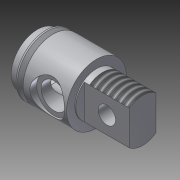
# Autodesk Inventor part: Rebuild Shooter NCDME075-0600 Cylinder Back Section
Saved by Autodesk Inventor 2014 SP1 (Build 180222100, 222)
## iProperties
Created: 2013-12-20
Part Number: Rebuild Shooter NCDME075-0600 Cylinder Back Section
Material: Aluminum 6061
Document SubType Name: Modeling
Designer: Moses
Mass: 18.68 g
Surface Area: 42.1842 cm^2
Volume: 6.893 cm^3
Density: 2.71 g/cm^3
Appearance: Aluminum - Flat
Author: Moses
Autodesk Inventor part; units mm, degrees
ref_plane "YZ Plane" through (0, 0, 0) normal (1, 0, 0) x (0, 1, 0)
ref_plane "XZ Plane" through (0, 0, 0) normal (0, 1, 0) x (-1, 0, 0)
sketch "Sketch1" plane through (0, 0, 0) normal (0, 0, 1) x (1, 0, 0)
  line L0 (0, 0) -> (35.3368, 0)
  line L1 (0, 10.922) -> (1.397, 9.525)
  line L2 (0, 10.922) -> (0.5388, 10.922)
  line L3 (0.5388, 10.922) -> (2.5708, 8.89)
  line L4 (2.5708, 8.89) -> (2.5708, 10.922)
  line L5 (2.5708, 10.922) -> (18.4458, 10.922)
  line L6 (18.4458, 10.922) -> (18.4458, 7.9248)
  line L7 (18.4458, 7.9248) -> (20.7318, 7.9248)
  line L8 (20.7318, 7.9248) -> (20.7318, 7.9375)
  line L9 (20.7318, 7.9375) -> (35.3368, 7.9375)
  line L10 (35.3368, 7.9375) -> (35.3368, 0)
  circle A0 centre (11.3338, 0) radius 4.7625
  circle A1 centre (27.0818, 0) radius 3.175
  line L11 (0, 10.922) -> (0, 0) construction
  line L12 (0.5388, 10.922) -> (2.5708, 10.922) construction
  line L13 (2.5708, 8.89) -> (2.5708, 7.9375) construction
  line L14 (1.397, 9.525) -> (0, 9.525)
  line L15 (0, 9.525) -> (0, 7.9375) construction
  line L16 (2.5708, 7.9375) -> (0, 7.9375)
  line L17 (0, 9.525) -> (0, 7.9375)
  line L18 (2.5708, 7.9375) -> (2.5708, 4.826)
  line L19 (2.5708, 4.826) -> (18.4458, 4.826)
  line L20 (18.4458, 4.826) -> (18.4458, 0)
  line L21 (18.4458, 7.9248) -> (18.4458, 4.826)
  line L22 (35.3368, 4.826) -> (18.4458, 4.826)
  line L23 (0, 9.525) -> (-3.175, 9.525)
  line L24 (-3.175, 9.525) -> (-3.175, 7.9375)
  line L25 (-3.175, 7.9375) -> (0, 7.9375)
  dimension "d1" = 21.844
  dimension "d2" = 9.525
  dimension "d4" = 2.286
  dimension "d5" = 6.35
  dimension "d6" = 8.636
  dimension "d8" = 15.8496
  dimension "d9" = 15.875
  dimension "d10" = 0.381
  dimension "d11" = 45
  dimension "d12" = 15.748
  dimension "d13" = 17.78
  dimension "d14" = 19.05
  dimension "d15" = 15.875
  dimension "d17" = 9.652
  dimension "d18" = 15.875
  dimension "d19" = 9.652
  dimension "d37" = 3.175
  dimension "d38" = 8.255
  constraints: 52 end point, 12 horizontal, 11 vertical, 7 point on line, 2 centre point, 1 parallel
  measures "d1" diameter of L5.end L0
  measures "d2" diameter of A0
  measures "d4" distance of L6.end L7.end
  measures "d5" diameter of A1
  measures "d6" horizontal distance of A1.centre L6.end
  measures "d8" diameter of L6.end L0
  measures "d9" distance of L4.end L5.end
  measures "d10" distance between parallel lines of L3 L1
  measures "d11" angle of L4 L3
  measures "d12" distance of A1.centre A0.centre
  measures "d13" diameter of L3.end L0
  measures "d14" diameter of L14.end L0
  measures "d15" diameter of L15.end L0
  measures "d17" diameter of L19 L0
  measures "d18" diameter of L9 L0
  measures "d19" diameter of L22.start L0
  measures "d37" distance of L14.end L23.end
  measures "d38" distance from line of L10 A1.centre
revolve "Revolution1" add sketch "Sketch1" angle 360 about axis through (0, 0, 0) along (1, 0, 0) picked at (27.874, 1.2084) contours L20 L22 L10 L0 A1 | A1 L0 | L19 L18 L16 L17 L14 L1 L2 L3 L4 L5 L6 L21 | L21 L7 L8 L9 L10 L22 | L25 L24 L23 L17
extrude "Extrusion2" cut sketch "Sketch1" along normal blind 25.4 contours A0 L0 | L0 A0
ref_plane "Work Plane1" through (10.5083, 0, 10.922) normal (0, 0, 1) x (1, 0, 0)
sketch "Sketch2" plane through (10.5083, 0, 10.922) normal (0, 0, 1) x (1, 0, 0)
  line L0 (0.8255, -4.7625) -> (0.8255, 0) construction
  circle A0 centre (0.8255, 0) radius 6.35
  point P0 (-10.5083, 0)
  dimension "d28" = 12.7
  dimension "d29" = 4.7625
  constraints: 2 end point, 1 centre point, 1 coincident, 1 vertical, 1 other
  measures "d28" diameter of A0
  measures "d29" distance of L0.start L0.end
extrude "Extrusion3" cut sketch "Sketch2" against normal blind 2.54
sketch "Sketch3" plane through (35.3368, 0, 0) normal (1, 0, 0) x (0, 0, -1)
  circle A0 centre (0, 0) radius 7.9375 projected
  line L0 (-4.826, 6.3019) -> (-4.826, -6.3019)
  line L1 (4.826, 6.3019) -> (4.826, -6.3019)
  dimension "d32" = 9.652
  constraints: 4 end point, 4 point on circle, 1 parallel, 1 vertical
  measures "d32" distance between parallel lines of L1 L0
extrude "Extrusion4" cut sketch "Sketch3" against normal blind 16.51 contours A0 L1 | L0 A0
extrude "Extrusion5" cut sketch "Sketch1" along normal through all both and the other way through all contours A1 L0 | L0 A1
thread "Thread1" size "5/8-11 UNC" class "2A" standard "ANSI Unified Screw Threads" full length
thread "Thread2" size "5/8-11 UNC" class "2A" standard "ANSI Unified Screw Threads" full length
equation "\"d17\" = d19"
body "Solid1"
